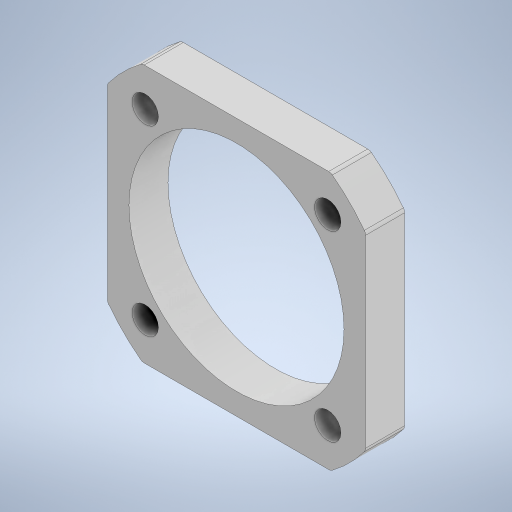
# Autodesk Inventor part: Ballscrew Spacer
Saved by Autodesk Inventor 2024 (Build 280153000, 153)
## iProperties
Created: 2024-12-31
Part Number: Ballscrew Spacer
Material: Generic
Document SubType Name: Modeling
Designer: Ishaan
Density: 1 g/cm^3
Appearance: Default
Author: Ishaan
Autodesk Inventor part; units mm, degrees
ref_plane "YZ Plane" through (0, 0, 0) normal (1, 0, 0) x (0, 1, 0)
ref_plane "XZ Plane" through (0, 0, 0) normal (0, 1, 0) x (-1, 0, 0)
ref_plane "XY Plane" through (0, 0, 0) normal (0, 0, 1) x (1, 0, 0)
sketch "Sketch1" plane through (0, 0, 0) normal (0, 0, 1) x (1, 0, 0)
  line L0 (21, -21) -> (-21, -21)
  line L1 (-21, -21) -> (-21, 21)
  line L2 (-21, 21) -> (21, 21)
  line L3 (21, 21) -> (21, -21)
  line L4 (21, -21) -> (-21, 21) construction
  line L5 (-21, -21) -> (21, 21) construction
  circle A0 centre (0, 0) radius 17.5
  circle A1 centre (0, 0) radius 26
  line L6 (0, 0) -> (-9.5671, 23.097) construction
  line L7 (0, 0) -> (0, 21) construction
  point P0 (-15.3297, 21)
  point P1 (-21, 15.3297)
  point P2 (-21, -15.3297)
  point P3 (-15.3297, -21)
  point P4 (15.3297, -21)
  point P5 (21, -15.3297)
  point P6 (21, 15.3297)
  point P7 (15.3297, 21)
  dimension "d0" = 42
  dimension "d1" = 42
  dimension "d2" = 35
  dimension "d3" = 52
  dimension "d4" = 25
  dimension "d5" = 22.5
  constraints: 16 end point, 3 midpoint, 2 centre point, 2 coincident, 2 parallel, 1 horizontal, 1 perpendicular
  measures "d0" distance of L1.end L2.end
  measures "d1" distance of L0.end L1.end
  measures "d2" diameter of A0
  measures "d3" diameter of A1
  measures "d4" distance of L6.start L6.end
  measures "d5" angle of L7 L6
extrude "Extrusion1" add sketch "Sketch1" along normal blind 6.35 contours L0 A1 L1 L2 L3
sketch "Sketch2" plane through (0, 0, 6.35) normal (0, 0, 1) x (1, 0, 0)
  line L0 (14.8492, -14.8492) -> (-14.8492, -14.8492)
  line L1 (-14.8492, -14.8492) -> (-14.8492, 14.8492)
  line L2 (-14.8492, 14.8492) -> (14.8492, 14.8492)
  line L3 (14.8492, 14.8492) -> (14.8492, -14.8492)
  line L4 (14.8492, -14.8492) -> (-14.8492, 14.8492) construction
  line L5 (-14.8492, -14.8492) -> (14.8492, 14.8492) construction
  point P0 (0, 0)
  dimension "d20" = 42
  constraints: 12 end point, 4 coincident, 2 midpoint, 2 parallel, 2 perpendicular, 1 horizontal
  measures "d20" distance of L0.start L1.end
hole "Hole2" at (-14.8492, 14.8492, 6.35) at (14.8492, 14.8492, 6.35) at (14.8492, -14.8492, 6.35) at (-14.8492, -14.8492, 6.35) direction (0, 0, -1) diameter 4.3 end through all
fillet "Fillet1" radius 1 8 edges at (15.3297, -21, 3.175) (21, -15.3297, 3.175) (-21, -15.3297, 3.175) (-15.3297, -21, 3.175) (21, 15.3297, 3.175) (15.3297, 21, 3.175) (-21, 15.3297, 3.175) (-15.3297, 21, 3.175)
body "Solid1"
